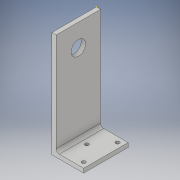
# Autodesk Inventor part: Suporte Direito
Saved by Autodesk Inventor 2017 (Build 210142000, 142)
## iProperties
Created: 2016-07-16
Part Number: Suporte Direito
Material: Generic
Document SubType Name: Modeling
Designer: mateu
Density: 1 g/cm^3
Appearance: Default
Author: mateu
Autodesk Inventor part; units mm, degrees
ref_plane "YZ Plane" through (0, 0, 0) normal (1, 0, 0) x (0, 1, 0)
ref_plane "XZ Plane" through (0, 0, 0) normal (0, 1, 0) x (-1, 0, 0)
ref_plane "XY Plane" through (0, 0, 0) normal (0, 0, 1) x (1, 0, 0)
sketch "Sketch1" plane through (0, 0, 0) normal (0, 0, 1) x (1, 0, 0)
  point P0 (0, 0)
sketch "Sketch2" plane through (0, 0, 0) normal (0, 0, 1) x (1, 0, 0)
  line L0 (0, 0) -> (0, -100)
  line L1 (0, -100) -> (30, -100)
  line L2 (30, -100) -> (30, -96)
  line L3 (30, -96) -> (4, -96)
  line L4 (4, -96) -> (4, 0)
  line L5 (4, 0) -> (0, 0)
  dimension "d0" = 100
  dimension "d1" = 30
  dimension "d2" = 4
  dimension "d3" = 26
  constraints: 12 end point, 4 perpendicular, 1 horizontal, 1 vertical
  measures "d0" distance of L0.start L0.end
  measures "d1" distance of L0.end L1.end
  measures "d2" distance of L1.end L2.end
  measures "d3" distance of L2.end L3.end
extrude "Extrusion1" add sketch "Sketch2" along normal blind 42
sketch "Sketch4" plane through (4, -96, 0) normal (0, 1, 0) x (1, 0, 0)
  line L0 (-4, -42) -> (26, -42) projected
  line L1 (-4, 0) -> (26, 0)
  line L2 (26, 0) -> (26, -42)
  line L3 (26, -42) -> (-4, -42)
  line L4 (-4, -42) -> (-4, 0)
  circle A0 centre (21, -37) radius 1.75
  circle A1 centre (21, -5) radius 1.75
  circle A2 centre (8, -21) radius 1.75
  dimension "d11" = 3.5
  dimension "d12" = 3.5
  dimension "d13" = 3.5
  dimension "d14" = 5
  dimension "d15" = 5
  dimension "d16" = 5
  dimension "d17" = 5
  dimension "d18" = 12
  dimension "d19" = 21
  constraints: 8 end point, 3 centre point, 2 parallel, 1 horizontal, 1 perpendicular
  measures "d11" diameter of A0
  measures "d12" diameter of A1
  measures "d13" diameter of A2
  measures "d14" distance from line of L2 A0.centre
  measures "d15" distance from line of L0 A0.centre
  measures "d16" distance from line of L2 A1.centre
  measures "d17" distance from line of L1 A1.centre
  measures "d18" distance from line of L4 A2.centre
  measures "d19" distance from line of L1 A2.centre
extrude "Extrusion3" cut sketch "Sketch4" against normal blind 4 contours A0 | A1 | A2
fillet "Fillet1" radius 3 1 edges at (4, -96, 21)
sketch "Sketch5" plane through (4, 0, 42) normal (1, 0, 0) x (0, 0, -1)
  line L0 (42, 0) -> (0, 0) projected
  line L1 (42, -100) -> (0, -100) projected
  line L2 (42, 0) -> (0, 0)
  line L3 (0, 0) -> (0, -100)
  line L4 (0, -100) -> (42, -100)
  line L5 (42, -100) -> (42, 0)
  circle A0 centre (21, -21) radius 6.8
  dimension "d23" = 13.6
  dimension "d24" = 21
  dimension "d25" = 21
  constraints: 8 end point, 2 parallel, 1 centre point, 1 horizontal, 1 perpendicular
  measures "d23" diameter of A0
  measures "d24" distance from line of L0 A0.centre
  measures "d25" distance from line of L3 A0.centre
extrude "Extrusion4" cut sketch "Sketch5" against normal blind 4 contours A0
body "Solid1"
